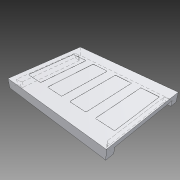
# Autodesk Inventor part: UNLHEP-14-01-P-017_GlueReservoit
Saved by Autodesk Inventor 2013 (Build 170138000, 138)
## iProperties
Created: 2014-01-23
Part Number: UNLHEP-14-01-P-017_GlueReservoit
Material: Aluminium 6061
Document SubType Name: Modeling
Designer: Frank Meier
Density: 2.71 g/cm^3
Mass: 683.997 g
Surface Area: 466.125 cm^2
Volume: 252.397 cm^3
Author: Frank Meier
Autodesk Inventor part; units mm, degrees
ref_plane "YZ Plane" through (0, 0, 0) normal (1, 0, 0) x (0, 1, 0)
ref_plane "XZ Plane" through (0, 0, 0) normal (0, 1, 0) x (-1, 0, 0)
ref_plane "XY Plane" through (0, 0, 0) normal (0, 0, 1) x (1, 0, 0)
sketch "Skizze1" plane through (0, 0, 0) normal (0, 0, 1) x (1, 0, 0)
  line L0 (-80, -60) -> (80, -60)
  line L1 (80, -60) -> (80, 60)
  line L2 (80, 60) -> (-80, 60)
  line L3 (-80, 60) -> (-80, -60)
  line L4 (-80, -60) -> (80, 60) construction
  line L5 (80, -60) -> (-80, 60) construction
  point P0 (0, 0)
  dimension "d0" = 160
  dimension "d1" = 120
  constraints: 12 end point, 2 midpoint, 2 parallel, 1 horizontal, 1 perpendicular
  measures "d0" distance of L1.end L2.end
  measures "d1" distance of L0.end L1.end
extrude "Extrusion1" add sketch "Skizze1" along normal blind 14
sketch "Skizze2" plane through (0, 0, 14) normal (0, 0, 1) x (1, 0, 0)
  line L0 (-80, -60) -> (80, -60) projected
  line L1 (-80, 60) -> (-80, -60) projected
  line L2 (-70, -37.5) -> (-45, -37.5)
  line L3 (-45, -37.5) -> (-45, 37.5)
  line L4 (-45, 37.5) -> (-70, 37.5)
  line L5 (-70, 37.5) -> (-70, -37.5)
  line L6 (-70, -37.5) -> (-45, 37.5) construction
  line L7 (-45, -37.5) -> (-70, 37.5) construction
  line L8 (-31.6667, -37.5) -> (-6.6667, -37.5)
  line L9 (-6.6667, -37.5) -> (-6.6667, 37.5)
  line L10 (-6.6667, 37.5) -> (-31.6667, 37.5)
  line L11 (-31.6667, 37.5) -> (-31.6667, -37.5)
  line L12 (-31.6667, -37.5) -> (-6.6667, 37.5) construction
  line L13 (-6.6667, -37.5) -> (-31.6667, 37.5) construction
  line L14 (6.6667, -37.5) -> (31.6667, -37.5)
  line L15 (31.6667, -37.5) -> (31.6667, 37.5)
  line L16 (31.6667, 37.5) -> (6.6667, 37.5)
  line L17 (6.6667, 37.5) -> (6.6667, -37.5)
  line L18 (6.6667, -37.5) -> (31.6667, 37.5) construction
  line L19 (31.6667, -37.5) -> (6.6667, 37.5) construction
  line L20 (45, -37.5) -> (70, -37.5)
  line L21 (70, -37.5) -> (70, 37.5)
  line L22 (70, 37.5) -> (45, 37.5)
  line L23 (45, 37.5) -> (45, -37.5)
  line L24 (45, -37.5) -> (70, 37.5) construction
  line L25 (70, -37.5) -> (45, 37.5) construction
  point P0 (-57.5, 0)
  point P1 (-19.1667, 0)
  point P2 (19.1667, 0)
  point P3 (57.5, 0)
  dimension "d4" = 25
  dimension "d5" = 75
  dimension "d6" = 10
  dimension "d7" = 60
  dimension "d47" = 38.3333
  constraints: 48 end point, 8 midpoint, 2 horizontal, 2 parallel, 1 perpendicular, 33 other
  measures "d4" distance of L3.end L4.end
  measures "d5" distance of L2.end L3.end
  measures "d6" distance between parallel lines of L1 L5
  measures "d7" distance from line of L0 point (-57.5, 0)
  measures "d47" distance of L2.start L8.start
extrude "Extrusion2" cut sketch "Skizze2" against normal blind 0.1
sketch "Skizze4" plane through (0, 0, 0) normal (0, 0, -1) x (-1, 0, 0)
  line L0 (80, 60) -> (80, -60) projected
  line L1 (-80, 60) -> (80, 60) projected
  line L2 (-80, -60) -> (-80, 60) projected
  line L3 (-80, 49) -> (-70, 49)
  line L4 (-70, 49) -> (-70, -49)
  line L5 (-70, -49) -> (-80, -49)
  line L6 (-80, -49) -> (-80, 49)
  line L7 (80, 49) -> (70, 49)
  line L8 (70, 49) -> (70, -49)
  line L9 (70, -49) -> (80, -49)
  line L10 (80, -49) -> (80, 49)
  point P0 (0, 0)
  dimension "d61" = 140
  dimension "d63" = 10
  dimension "d64" = 11
  dimension "d65" = 98
  constraints: 16 end point, 4 parallel, 2 collinear, 2 horizontal, 2 perpendicular, 2 point on line
  measures "d61" distance between parallel lines of L8 L4
  measures "d63" distance of L4.end L5.end
  measures "d64" distance between parallel lines of L1 L3
  measures "d65" distance between parallel lines of L5 L3
extrude "Extrusion3" cut sketch "Skizze4" against normal blind 8
fillet "Rundung1" radius 2 4 edges at (-70, -49, 4) (-70, 49, 4) (70, 49, 4) (70, -49, 4)
fillet "Rundung2" radius 1 1 edges at (-70, 37.5, 13.95)
fillet "Rundung3" radius 1 1 edges at (-45, 37.5, 13.95)
fillet "Rundung4" radius 1 14 edges at (-31.6667, 37.5, 13.95) (-70, -37.5, 13.95) (-6.6667, -37.5, 13.95) (-31.6667, -37.5, 13.95) (-45, -37.5, 13.95) (6.6667, -37.5, 13.95) (31.6667, -37.5, 13.95) (45, -37.5, 13.95) (70, -37.5, 13.95) (70, 37.5, 13.95) (-6.6667, 37.5, 13.95) (6.6667, 37.5, 13.95) (31.6667, 37.5, 13.95) (45, 37.5, 13.95)
